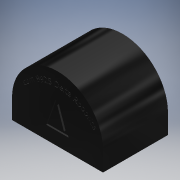
# Autodesk Inventor part: wheel cover
Saved by Autodesk Inventor 2019 (Build 230136000, 136)
## iProperties
Part Number: wheel cover
Material: Generic
Document SubType Name: Modeling
Designer: Delta
Appearance: Default(1)
Author: Delta
Autodesk Inventor part; units mm, degrees
ref_plane "YZ Plane" through (0, 0, 0) normal (1, 0, 0) x (0, 1, 0)
ref_plane "XZ Plane" through (0, 0, 0) normal (0, 1, 0) x (-1, 0, 0)
ref_plane "XY Plane" through (0, 0, 0) normal (0, 0, 1) x (1, 0, 0)
sketch "Sketch2" plane through (0, 0, 0) normal (0, 0, 1) x (1, 0, 0)
  circle A0 centre (0, 0) radius 44.45
  line L0 (44.45, 0) -> (-44.45, 0)
  dimension "d3" = 88.9
  constraints: 2 end point, 2 point on circle, 1 centre point, 1 coincident, 1 horizontal
  measures "d3" diameter of A0
extrude "Extrusion2" add sketch "Sketch2" along normal blind 63.5 contours L0 A0 picked at (-1.5488, 26.7885)
shell "Shell2" thickness 3.175 removed faces 1 at (4.5786, 14.0915, 0)
sketch "Sketch3" plane through (-44.45, 0, 0) normal (0, -1, 0) x (1, 0, 0)
  line L0 (3.2973, 0) -> (3.2973, 60.325) projected
  line L1 (3.2973, 60.325) -> (85.6027, 60.325) projected
  line L2 (85.6027, 0) -> (85.6027, 60.325) projected
  line L3 (0, 0) -> (88.9, 0) projected
  point P0 (44.45, 0)
extrude "Extrusion3" cut sketch "Sketch3" against normal blind 3.175
sketch "Sketch8" plane through (-44.45, 0, 63.5) normal (0, -1, 0) x (1, 0, 0)
  line L0 (3.2973, -63.5) -> (3.2973, -3.175) projected
  line L1 (3.2973, -3.175) -> (85.6027, -3.175) projected
  line L2 (85.6027, -3.175) -> (85.6027, -63.5) projected
  line L3 (85.6027, -63.5) -> (88.9, -63.5) projected
  line L4 (88.9, -63.5) -> (88.9, 0) projected
  line L5 (0, 0) -> (88.9, 0) projected
  line L6 (0, -63.5) -> (0, 0) projected
  line L7 (0, -63.5) -> (3.2973, -63.5) projected
  point P0 (44.45, -63.5)
extrude "Extrusion6" add sketch "Sketch8" along normal blind 19.05
sketch "Sketch15" plane through (0, 0, 63.5) normal (0, 0, 1) x (1, 0, 0)
  line L0 (-19.05, 19.05) -> (19.05, 19.05) construction
  line L1 (19.05, 19.05) -> (19.05, -6.35) construction
  line L2 (19.05, -6.35) -> (-19.05, -6.35) construction
  line L3 (-19.05, -6.35) -> (-19.05, 19.05) construction
  line L4 (44.45, -17.78) -> (44.45, 0) projected
  line L5 (-44.45, 0) -> (-44.45, -17.78) projected
  line L6 (-43.18, -19.05) -> (43.18, -19.05) projected
  line L7 (10.8166, -6.35) -> (-11.1459, -6.35)
  line L8 (-11.1459, -6.35) -> (-2.2539, 19.05)
  line L9 (-2.2539, 19.05) -> (1.9246, 19.05)
  line L10 (1.9246, 19.05) -> (10.8166, -6.35)
  line L11 (6.2677, -3.4271) -> (-0.2573, 15.7155)
  line L12 (-0.2573, 15.7155) -> (-6.7411, -3.4271)
  line L13 (-6.7411, -3.4271) -> (6.2677, -3.4271)
  point P0 (0, 0)
  dimension "d55" = 25.4
  dimension "d56" = 25.4
  dimension "d57" = 12.7
  dimension "d58" = 38.1
  constraints: 2 other
  measures "d55" distance between parallel lines of L4 L1
  measures "d56" distance between parallel lines of L5 L3
  measures "d57" distance between parallel lines of L6 L2
  measures "d58" distance between parallel lines of L6 L0
extrude "Extrusion10" cut sketch "Sketch15" against normal blind 1.5875
sketch "Sketch16" plane through (0, 0, 63.5) normal (0, 0, 1) x (1, 0, 0)
  line L0 (-44.45, 0) -> (-44.45, -17.78) projected
  line L1 (-43.18, 41.275) -> (-43.18, -17.78) projected
  arc A0 (42.9782, -8.89) -> (-43.18, -8.89) centre (-0.1009, -13.0404) ccw
  line L2 (-43.18, -8.89) -> (42.9782, -8.89) construction
  line L3 (-43.18, -8.89) -> (42.9782, -8.89) construction
  line L4 (-33.5603, 14.4116) -> (-37.0005, 17.2799)
  line L5 (-37.0005, 17.2799) -> (-38.0919, 15.9708)
  line L6 (-38.0919, 15.9708) -> (-38.5535, 16.3557)
  line L7 (-38.5535, 16.3557) -> (-35.9384, 19.4923)
  line L8 (-35.9384, 19.4923) -> (-35.4767, 19.1074)
  line L9 (-35.4767, 19.1074) -> (-36.5681, 17.7984)
  line L10 (-36.5681, 17.7984) -> (-33.128, 14.9302)
  line L11 (-33.128, 14.9302) -> (-33.5603, 14.4116)
  spline S0 degree 2 poles (-30.4682, 17.6755) (-31.1139, 17.0287) (-32.549, 17.0421) (-33.219, 17.7111) knots 0 0 0 1 2 2 2
  spline S1 degree 2 poles (-33.219, 17.7111) (-33.8774, 18.3684) (-33.9689, 19.8384) (-33.4134, 20.3948) knots 0 0 0 1 2 2 2
  spline S2 degree 2 poles (-33.4134, 20.3948) (-33.1632, 20.6454) (-32.6307, 20.8874) (-32.3338, 20.876) knots 0 0 0 1 2 2 2
  spline S3 degree 2 poles (-32.3338, 20.876) (-32.034, 20.8675) (-31.4341, 20.5769) (-31.1107, 20.2541) knots 0 0 0 1 2 2 2
  line L12 (-31.1107, 20.2541) -> (-30.863, 20.0068)
  line L13 (-30.863, 20.0068) -> (-32.7274, 18.1394)
  spline S4 degree 2 poles (-32.7274, 18.1394) (-32.2584, 17.6711) (-31.289, 17.6457) (-30.8702, 18.0652) knots 0 0 0 1 2 2 2
  spline S5 degree 2 poles (-30.8702, 18.0652) (-30.7219, 18.2138) (-30.5009, 18.5691) (-30.437, 18.738) knots 0 0 0 1 2 2 2
  spline S6 degree 2 poles (-30.437, 18.738) (-30.3731, 18.9185) (-30.3064, 19.1893) (-30.2977, 19.2912) knots 0 0 0 1 2 2 2
  line L14 (-30.2977, 19.2912) -> (-30.2716, 19.3174)
  line L15 (-30.2716, 19.3174) -> (-29.7763, 18.823)
  spline S7 degree 2 poles (-29.7763, 18.823) (-29.8228, 18.7123) (-29.9681, 18.3804) (-30.0349, 18.2609) knots 0 0 0 1 2 2 2
  spline S8 degree 2 poles (-30.0349, 18.2609) (-30.1279, 18.092) (-30.3053, 17.8386) (-30.4682, 17.6755) knots 0 0 0 1 2 2 2
  spline S9 degree 2 poles (-31.6518, 19.9101) (-31.8412, 20.0875) (-32.1848, 20.2794) (-32.3479, 20.2967) knots 0 0 0 1 2 2 2
  spline S10 degree 2 poles (-32.3479, 20.2967) (-32.5284, 20.3198) (-32.8834, 20.1798) (-33.0666, 19.9963) knots 0 0 0 1 2 2 2
  spline S11 degree 2 poles (-33.0666, 19.9963) (-33.247, 19.8157) (-33.3922, 19.4546) (-33.392, 19.245) knots 0 0 0 1 2 2 2
  spline S12 degree 2 poles (-33.392, 19.245) (-33.386, 19.0354) (-33.2315, 18.6717) (-33.0741, 18.4855) knots 0 0 0 1 2 2 2
  line L16 (-33.0741, 18.4855) -> (-31.6518, 19.9101)
  spline S13 degree 2 poles (-27.712, 20.8168) (-27.7346, 20.7223) (-27.803, 20.3951) (-27.8575, 20.2682) knots 0 0 0 1 2 2 2
  spline S14 degree 2 poles (-27.8575, 20.2682) (-27.928, 20.0901) (-28.1091, 19.8132) (-28.3292, 19.6273) knots 0 0 0 1 2 2 2
  spline S15 degree 2 poles (-28.3292, 19.6273) (-28.5085, 19.4758) (-28.9466, 19.3374) (-29.1729, 19.3565) knots 0 0 0 1 2 2 2
  spline S16 degree 2 poles (-29.1729, 19.3565) (-29.3902, 19.3777) (-29.8292, 19.6104) (-29.9939, 19.8054) knots 0 0 0 1 2 2 2
  spline S17 degree 2 poles (-29.9939, 19.8054) (-30.249, 20.1073) (-30.3555, 20.7501) (-30.1824, 21.1066) knots 0 0 0 1 2 2 2
  spline S18 degree 2 poles (-30.1824, 21.1066) (-30.0327, 21.427) (-29.4377, 22.0751) (-29.0695, 22.4238) knots 0 0 0 1 2 2 2
  line L17 (-29.0695, 22.4238) -> (-29.1492, 22.5182)
  spline S19 degree 2 poles (-29.1492, 22.5182) (-29.2926, 22.688) (-29.5744, 22.8111) (-29.7192, 22.7911) knots 0 0 0 1 2 2 2
  spline S20 degree 2 poles (-29.7192, 22.7911) (-29.8641, 22.7712) (-30.1664, 22.5804) (-30.311, 22.4582) knots 0 0 0 1 2 2 2
  spline S21 degree 2 poles (-30.311, 22.4582) (-30.4809, 22.3148) (-30.855, 21.8263) (-31.0022, 21.5349) knots 0 0 0 1 2 2 2
  line L18 (-31.0022, 21.5349) -> (-31.0305, 21.511)
  line L19 (-31.0305, 21.511) -> (-31.4529, 22.011)
  spline S22 degree 2 poles (-31.4529, 22.011) (-31.3496, 22.163) (-30.9229, 22.685) (-30.6745, 22.8949) knots 0 0 0 1 2 2 2
  spline S23 degree 2 poles (-30.6745, 22.8949) (-30.3726, 23.1499) (-29.8809, 23.4036) (-29.6138, 23.4191) knots 0 0 0 1 2 2 2
  spline S24 degree 2 poles (-29.6138, 23.4191) (-29.3525, 23.435) (-28.8738, 23.1873) (-28.6427, 22.9137) knots 0 0 0 1 2 2 2
  line L20 (-28.6427, 22.9137) -> (-26.9611, 20.923)
  line L21 (-26.9611, 20.923) -> (-27.4517, 20.5086)
  line L22 (-27.4517, 20.5086) -> (-27.712, 20.8168)
  line L23 (-28.0574, 21.2257) -> (-28.7401, 22.0339)
  spline S25 degree 2 poles (-28.7401, 22.0339) (-28.9029, 21.8694) (-29.3892, 21.367) (-29.5134, 21.1759) knots 0 0 0 1 2 2 2
  spline S26 degree 2 poles (-29.5134, 21.1759) (-29.6579, 20.9514) (-29.7028, 20.4878) (-29.5168, 20.2677) knots 0 0 0 1 2 2 2
  spline S27 degree 2 poles (-29.5168, 20.2677) (-29.3043, 20.0161) (-28.8061, 20.0004) (-28.5356, 20.2289) knots 0 0 0 1 2 2 2
  spline S28 degree 2 poles (-28.5356, 20.2289) (-28.3061, 20.4228) (-28.096, 20.9397) (-28.0574, 21.2257) knots 0 0 0 1 2 2 2
  line L24 (-22.6902, 23.9217) -> (-23.9204, 25.7535)
  spline S29 degree 2 poles (-23.9204, 25.7535) (-24.0673, 25.9722) (-24.3516, 26.3218) (-24.4751, 26.3876) knots 0 0 0 1 2 2 2
  spline S30 degree 2 poles (-24.4751, 26.3876) (-24.6056, 26.4636) (-24.8875, 26.433) (-25.0686, 26.3113) knots 0 0 0 1 2 2 2
  spline S31 degree 2 poles (-25.0686, 26.3113) (-25.2326, 26.2012) (-25.4732, 25.7471) (-25.5428, 25.4226) knots 0 0 0 1 2 2 2
  spline S32 degree 2 poles (-25.5428, 25.4226) (-25.5073, 25.377) (-25.4109, 25.2483) (-25.3513, 25.1595) knots 0 0 0 1 2 2 2
  line L25 (-25.3513, 25.1595) -> (-23.9512, 23.0748)
  line L26 (-23.9512, 23.0748) -> (-24.4844, 22.7167)
  line L27 (-24.4844, 22.7167) -> (-25.7146, 24.5485)
  spline S33 degree 2 poles (-25.7146, 24.5485) (-25.8615, 24.7672) (-26.1458, 25.1168) (-26.2693, 25.1826) knots 0 0 0 1 2 2 2
  spline S34 degree 2 poles (-26.2693, 25.1826) (-26.3998, 25.2587) (-26.6817, 25.228) (-26.8628, 25.1064) knots 0 0 0 1 2 2 2
  spline S35 degree 2 poles (-26.8628, 25.1064) (-27.0337, 24.9916) (-27.2684, 24.5215) (-27.3337, 24.2347) knots 0 0 0 1 2 2 2
  line L28 (-27.3337, 24.2347) -> (-25.7454, 21.8698)
  line L29 (-25.7454, 21.8698) -> (-26.2786, 21.5118)
  line L30 (-26.2786, 21.5118) -> (-28.4039, 24.6764)
  line L31 (-28.4039, 24.6764) -> (-27.8707, 25.0344)
  line L32 (-27.8707, 25.0344) -> (-27.6366, 24.6859)
  spline S36 degree 2 poles (-27.6366, 24.6859) (-27.5682, 25.0343) (-27.3118, 25.5387) (-27.0658, 25.704) knots 0 0 0 1 2 2 2
  spline S37 degree 2 poles (-27.0658, 25.704) (-26.7855, 25.8922) (-26.1794, 25.9273) (-25.8715, 25.7126) knots 0 0 0 1 2 2 2
  spline S38 degree 2 poles (-25.8715, 25.7126) (-25.8102, 26.1455) (-25.5382, 26.7299) (-25.2716, 26.9089) knots 0 0 0 1 2 2 2
  spline S39 degree 2 poles (-25.2716, 26.9089) (-25.0665, 27.0466) (-24.6467, 27.1451) (-24.4273, 27.0842) knots 0 0 0 1 2 2 2
  spline S40 degree 2 poles (-24.4273, 27.0842) (-24.2044, 27.0256) (-23.7751, 26.6891) (-23.5571, 26.3644) knots 0 0 0 1 2 2 2
  line L33 (-23.5571, 26.3644) -> (-22.157, 24.2797)
  line L34 (-22.157, 24.2797) -> (-22.6902, 23.9217)
  spline S41 degree 2 poles (-21.0664, 28.7312) (-21.2291, 29.0868) (-21.2678, 29.7845) (-21.1634, 30.0904) knots 0 0 0 1 2 2 2
  spline S42 degree 2 poles (-21.1634, 30.0904) (-21.0667, 30.3836) (-20.6135, 30.8673) (-20.329, 30.9975) knots 0 0 0 1 2 2 2
  spline S43 degree 2 poles (-20.329, 30.9975) (-20.0109, 31.1432) (-19.3966, 31.1663) (-19.1132, 31.0516) knots 0 0 0 1 2 2 2
  spline S44 degree 2 poles (-19.1132, 31.0516) (-18.7571, 30.9067) (-18.1181, 30.2032) (-17.8285, 29.5706) knots 0 0 0 1 2 2 2
  spline S45 degree 2 poles (-17.8285, 29.5706) (-17.5664, 28.9979) (-17.3551, 27.854) (-17.45, 27.3986) knots 0 0 0 1 2 2 2
  spline S46 degree 2 poles (-17.45, 27.3986) (-17.5512, 26.9176) (-18.1268, 26.1968) (-18.6733, 25.9466) knots 0 0 0 1 2 2 2
  spline S47 degree 2 poles (-18.6733, 25.9466) (-18.7968, 25.8901) (-19.0895, 25.7878) (-19.2264, 25.7704) knots 0 0 0 1 2 2 2
  line L35 (-19.2264, 25.7704) -> (-19.4989, 26.3655)
  line L36 (-19.4989, 26.3655) -> (-19.469, 26.3792)
  spline S48 degree 2 poles (-19.469, 26.3792) (-19.3698, 26.3703) (-19.0044, 26.4425) (-18.836, 26.5196) knots 0 0 0 1 2 2 2
  spline S49 degree 2 poles (-18.836, 26.5196) (-18.2296, 26.7972) (-17.9038, 27.9152) (-18.1944, 28.6787) knots 0 0 0 1 2 2 2
  spline S50 degree 2 poles (-18.1944, 28.6787) (-18.3644, 28.3971) (-18.7433, 28.038) (-19.0091, 27.9164) knots 0 0 0 1 2 2 2
  spline S51 degree 2 poles (-19.0091, 27.9164) (-19.2636, 27.7998) (-19.738, 27.7185) (-20.025, 27.7818) knots 0 0 0 1 2 2 2
  spline S52 degree 2 poles (-20.025, 27.7818) (-20.3594, 27.8596) (-20.8796, 28.3232) (-21.0664, 28.7312) knots 0 0 0 1 2 2 2
  spline S53 degree 2 poles (-18.517, 29.4229) (-18.7312, 29.8908) (-19.1742, 30.4034) (-19.4013, 30.4941) knots 0 0 0 1 2 2 2
  spline S54 degree 2 poles (-19.4013, 30.4941) (-19.6046, 30.5821) (-19.9367, 30.5659) (-20.1014, 30.4905) knots 0 0 0 1 2 2 2
  spline S55 degree 2 poles (-20.1014, 30.4905) (-20.4832, 30.3157) (-20.686, 29.5619) (-20.4495, 29.0453) knots 0 0 0 1 2 2 2
  spline S56 degree 2 poles (-20.4495, 29.0453) (-20.3158, 28.7534) (-19.9931, 28.4438) (-19.7667, 28.3845) knots 0 0 0 1 2 2 2
  spline S57 degree 2 poles (-19.7667, 28.3845) (-19.6023, 28.342) (-19.2775, 28.4137) (-19.1053, 28.4926) knots 0 0 0 1 2 2 2
  spline S58 degree 2 poles (-19.1053, 28.4926) (-18.9069, 28.5834) (-18.5137, 28.9309) (-18.3946, 29.1258) knots 0 0 0 1 2 2 2
  spline S59 degree 2 poles (-18.3946, 29.1258) (-18.4114, 29.1724) (-18.4742, 29.3293) (-18.517, 29.4229) knots 0 0 0 1 2 2 2
  spline S60 degree 2 poles (-17.313, 30.4126) (-17.4439, 30.7811) (-17.4211, 31.4795) (-17.2901, 31.775) knots 0 0 0 1 2 2 2
  spline S61 degree 2 poles (-17.2901, 31.775) (-17.1681, 32.0586) (-16.6741, 32.5006) (-16.3793, 32.6053) knots 0 0 0 1 2 2 2
  spline S62 degree 2 poles (-16.3793, 32.6053) (-16.0495, 32.7224) (-15.4357, 32.6914) (-15.1634, 32.5522) knots 0 0 0 1 2 2 2
  spline S63 degree 2 poles (-15.1634, 32.5522) (-14.8214, 32.3766) (-14.2468, 31.6196) (-14.0139, 30.9641) knots 0 0 0 1 2 2 2
  spline S64 degree 2 poles (-14.0139, 30.9641) (-13.8031, 30.3705) (-13.6932, 29.2125) (-13.8278, 28.7672) knots 0 0 0 1 2 2 2
  spline S65 degree 2 poles (-13.8278, 28.7672) (-13.9709, 28.297) (-14.6076, 27.6296) (-15.174, 27.4284) knots 0 0 0 1 2 2 2
  spline S66 degree 2 poles (-15.174, 27.4284) (-15.302, 27.383) (-15.6026, 27.3068) (-15.7405, 27.3015) knots 0 0 0 1 2 2 2
  line L37 (-15.7405, 27.3015) -> (-15.9596, 27.9183)
  line L38 (-15.9596, 27.9183) -> (-15.9285, 27.9293)
  spline S67 degree 2 poles (-15.9285, 27.9293) (-15.8305, 27.9117) (-15.4602, 27.9515) (-15.2857, 28.0135) knots 0 0 0 1 2 2 2
  spline S68 degree 2 poles (-15.2857, 28.0135) (-14.6572, 28.2367) (-14.2344, 29.3217) (-14.4568, 30.1078) knots 0 0 0 1 2 2 2
  spline S69 degree 2 poles (-14.4568, 30.1078) (-14.6508, 29.8422) (-15.0598, 29.5179) (-15.3353, 29.42) knots 0 0 0 1 2 2 2
  spline S70 degree 2 poles (-15.3353, 29.42) (-15.5991, 29.3263) (-16.0788, 29.287) (-16.3591, 29.3753) knots 0 0 0 1 2 2 2
  spline S71 degree 2 poles (-16.3591, 29.3753) (-16.6854, 29.4822) (-17.1628, 29.9898) (-17.313, 30.4126) knots 0 0 0 1 2 2 2
  spline S72 degree 2 poles (-14.7127, 30.8775) (-14.885, 31.3624) (-15.2811, 31.9119) (-15.4994, 32.0222) knots 0 0 0 1 2 2 2
  spline S73 degree 2 poles (-15.4994, 32.0222) (-15.6942, 32.1278) (-16.0265, 32.1408) (-16.1971, 32.0802) knots 0 0 0 1 2 2 2
  spline S74 degree 2 poles (-16.1971, 32.0802) (-16.5928, 31.9397) (-16.861, 31.2066) (-16.6709, 30.6712) knots 0 0 0 1 2 2 2
  spline S75 degree 2 poles (-16.6709, 30.6712) (-16.5634, 30.3687) (-16.2691, 30.032) (-16.0488, 29.9529) knots 0 0 0 1 2 2 2
  spline S76 degree 2 poles (-16.0488, 29.9529) (-15.8888, 29.8962) (-15.559, 29.9391) (-15.3805, 30.0025) knots 0 0 0 1 2 2 2
  spline S77 degree 2 poles (-15.3805, 30.0025) (-15.1749, 30.0755) (-14.7526, 30.3871) (-14.6169, 30.5708) knots 0 0 0 1 2 2 2
  spline S78 degree 2 poles (-14.6169, 30.5708) (-14.6295, 30.6187) (-14.6783, 30.7805) (-14.7127, 30.8775) knots 0 0 0 1 2 2 2
  line L39 (-9.3987, 29.2577) -> (-12.4316, 28.4728)
  line L40 (-12.4316, 28.4728) -> (-12.6121, 29.1702)
  spline S79 degree 2 poles (-12.6121, 29.1702) (-12.3647, 29.5617) (-11.9304, 30.2822) (-11.7308, 30.6613) knots 0 0 0 1 2 2 2
  spline S80 degree 2 poles (-11.7308, 30.6613) (-11.3287, 31.4244) (-11.1101, 32.2719) (-11.2122, 32.6665) knots 0 0 0 1 2 2 2
  spline S81 degree 2 poles (-11.2122, 32.6665) (-11.2659, 32.8737) (-11.4739, 33.1516) (-11.6152, 33.2213) knots 0 0 0 1 2 2 2
  spline S82 degree 2 poles (-11.6152, 33.2213) (-11.7566, 33.291) (-12.0853, 33.3123) (-12.2686, 33.2648) knots 0 0 0 1 2 2 2
  spline S83 degree 2 poles (-12.2686, 33.2648) (-12.4439, 33.2194) (-12.7799, 33.0389) (-12.9258, 32.9289) knots 0 0 0 1 2 2 2
  spline S84 degree 2 poles (-12.9258, 32.9289) (-13.0508, 32.837) (-13.2686, 32.6105) (-13.3339, 32.5341) knots 0 0 0 1 2 2 2
  line L41 (-13.3339, 32.5341) -> (-13.3698, 32.5248)
  line L42 (-13.3698, 32.5248) -> (-13.5513, 33.2262)
  spline S85 degree 2 poles (-13.5513, 33.2262) (-13.3738, 33.3785) (-12.6951, 33.7625) (-12.3683, 33.8471) knots 0 0 0 1 2 2 2
  spline S86 degree 2 poles (-12.3683, 33.8471) (-11.6788, 34.0256) (-10.7129, 33.4974) (-10.552, 32.8757) knots 0 0 0 1 2 2 2
  spline S87 degree 2 poles (-10.552, 32.8757) (-10.4767, 32.5847) (-10.4863, 32.0634) (-10.5523, 31.8253) knots 0 0 0 1 2 2 2
  spline S88 degree 2 poles (-10.5523, 31.8253) (-10.6161, 31.5791) (-10.8535, 31.0669) (-10.9922, 30.8141) knots 0 0 0 1 2 2 2
  spline S89 degree 2 poles (-10.9922, 30.8141) (-11.2154, 30.3949) (-11.7888, 29.4726) (-11.9613, 29.2026) knots 0 0 0 1 2 2 2
  line L43 (-11.9613, 29.2026) -> (-9.5462, 29.8277)
  line L44 (-9.5462, 29.8277) -> (-9.3987, 29.2577)
  spline S90 degree 2 poles (-5.9624, 31.4943) (-5.9022, 31.1329) (-6.0307, 30.4771) (-6.2039, 30.2145) knots 0 0 0 1 2 2 2
  spline S91 degree 2 poles (-6.2039, 30.2145) (-6.3772, 29.9519) (-6.9626, 29.583) (-7.3524, 29.518) knots 0 0 0 1 2 2 2
  spline S92 degree 2 poles (-7.3524, 29.518) (-7.7097, 29.4584) (-8.4345, 29.5003) (-8.7114, 29.5835) knots 0 0 0 1 2 2 2
  line L45 (-8.7114, 29.5835) -> (-8.8299, 30.2941)
  line L46 (-8.8299, 30.2941) -> (-8.7811, 30.3023)
  spline S93 degree 2 poles (-8.7811, 30.3023) (-8.6945, 30.2583) (-8.3818, 30.1602) (-8.1964, 30.1243) knots 0 0 0 1 2 2 2
  spline S94 degree 2 poles (-8.1964, 30.1243) (-7.9859, 30.0885) (-7.6441, 30.0662) (-7.437, 30.1007) knots 0 0 0 1 2 2 2
  spline S95 degree 2 poles (-7.437, 30.1007) (-7.234, 30.1346) (-6.8767, 30.3444) (-6.765, 30.5258) knots 0 0 0 1 2 2 2
  spline S96 degree 2 poles (-6.765, 30.5258) (-6.6642, 30.697) (-6.6006, 31.1166) (-6.6453, 31.3846) knots 0 0 0 1 2 2 2
  spline S97 degree 2 poles (-6.6453, 31.3846) (-6.69, 31.6526) (-6.8931, 31.9693) (-7.0501, 32.06) knots 0 0 0 1 2 2 2
  spline S98 degree 2 poles (-7.0501, 32.06) (-7.2132, 32.1622) (-7.6531, 32.1973) (-7.9089, 32.1547) knots 0 0 0 1 2 2 2
  spline S99 degree 2 poles (-7.9089, 32.1547) (-8.185, 32.1086) (-8.719, 31.9319) (-8.8794, 31.8676) knots 0 0 0 1 2 2 2
  line L47 (-8.8794, 31.8676) -> (-9.3101, 34.4502)
  line L48 (-9.3101, 34.4502) -> (-6.561, 34.9086)
  line L49 (-6.561, 34.9086) -> (-6.4628, 34.3198)
  line L50 (-6.4628, 34.3198) -> (-8.5662, 33.9691)
  line L51 (-8.5662, 33.9691) -> (-8.3435, 32.6331)
  spline S100 degree 2 poles (-8.3435, 32.6331) (-8.2244, 32.6697) (-7.9909, 32.7211) (-7.8934, 32.7374) knots 0 0 0 1 2 2 2
  spline S101 degree 2 poles (-7.8934, 32.7374) (-7.5077, 32.8017) (-6.9547, 32.7645) (-6.6799, 32.6184) knots 0 0 0 1 2 2 2
  spline S102 degree 2 poles (-6.6799, 32.6184) (-6.4011, 32.4729) (-6.0383, 31.9491) (-5.9624, 31.4943) knots 0 0 0 1 2 2 2
  spline S103 degree 2 poles (1.3105, 32.8027) (1.3218, 32.1071) (0.7759, 30.9784) (0.3076, 30.658) knots 0 0 0 1 2 2 2
  spline S104 degree 2 poles (0.3076, 30.658) (-0.0754, 30.4089) (-0.8671, 30.2314) (-1.4846, 30.2214) knots 0 0 0 1 2 2 2
  line L52 (-1.4846, 30.2214) -> (-2.6536, 30.2026)
  line L53 (-2.6536, 30.2026) -> (-2.7355, 35.2819)
  line L54 (-2.7355, 35.2819) -> (-1.5789, 35.3006)
  spline S105 degree 2 poles (-1.5789, 35.3006) (-0.8627, 35.3121) (-0.0442, 35.1112) (0.247, 34.9265) knots 0 0 0 1 2 2 2
  spline S106 degree 2 poles (0.247, 34.9265) (0.742, 34.6093) (1.2986, 33.5437) (1.3105, 32.8027) knots 0 0 0 1 2 2 2
  spline S107 degree 2 poles (0.6066, 32.7996) (0.5971, 33.3841) (0.1969, 34.2052) (-0.1897, 34.4337) knots 0 0 0 1 2 2 2
  spline S108 degree 2 poles (-0.1897, 34.4337) (-0.464, 34.5898) (-1.0796, 34.724) (-1.5365, 34.7166) knots 0 0 0 1 2 2 2
  line L55 (-1.5365, 34.7166) -> (-2.051, 34.7083)
  line L56 (-2.051, 34.7083) -> (-1.9879, 30.798)
  line L57 (-1.9879, 30.798) -> (-1.4734, 30.8063)
  spline S109 degree 2 poles (-1.4734, 30.8063) (-1.0248, 30.8135) (-0.3479, 30.9685) (-0.0753, 31.1664) knots 0 0 0 1 2 2 2
  spline S110 degree 2 poles (-0.0753, 31.1664) (0.2749, 31.4109) (0.6161, 32.2069) (0.6066, 32.7996) knots 0 0 0 1 2 2 2
  spline S111 degree 2 poles (3.6748, 29.9873) (2.7639, 30.0612) (1.8456, 31.1642) (1.9222, 32.1079) knots 0 0 0 1 2 2 2
  spline S112 degree 2 poles (1.9222, 32.1079) (1.9975, 33.0352) (3.0592, 34.0559) (3.8429, 33.9923) knots 0 0 0 1 2 2 2
  spline S113 degree 2 poles (3.8429, 33.9923) (4.1958, 33.9637) (4.7249, 33.7142) (4.9083, 33.4804) knots 0 0 0 1 2 2 2
  spline S114 degree 2 poles (4.9083, 33.4804) (5.0958, 33.2463) (5.2623, 32.6009) (5.2253, 32.1454) knots 0 0 0 1 2 2 2
  line L58 (5.2253, 32.1454) -> (5.197, 31.7966)
  line L59 (5.197, 31.7966) -> (2.5669, 32.0101)
  spline S115 degree 2 poles (2.5669, 32.0101) (2.5133, 31.3495) (3.121, 30.5939) (3.7119, 30.546) knots 0 0 0 1 2 2 2
  spline S116 degree 2 poles (3.7119, 30.546) (3.9211, 30.529) (4.335, 30.5904) (4.5051, 30.6509) knots 0 0 0 1 2 2 2
  spline S117 degree 2 poles (4.5051, 30.6509) (4.6841, 30.719) (4.9338, 30.8433) (5.0171, 30.9026) knots 0 0 0 1 2 2 2
  line L60 (5.0171, 30.9026) -> (5.054, 30.8996)
  line L61 (5.054, 30.8996) -> (4.9974, 30.202)
  spline S118 degree 2 poles (4.9974, 30.202) (4.8829, 30.1659) (4.5358, 30.0619) (4.4015, 30.0356) knots 0 0 0 1 2 2 2
  spline S119 degree 2 poles (4.4015, 30.0356) (4.2125, 29.9973) (3.9046, 29.9686) (3.6748, 29.9873) knots 0 0 0 1 2 2 2
  spline S120 degree 2 poles (4.613, 32.3355) (4.6258, 32.5947) (4.5497, 32.9809) (4.4575, 33.1164) knots 0 0 0 1 2 2 2
  spline S121 degree 2 poles (4.4575, 33.1164) (4.3583, 33.269) (4.0219, 33.4491) (3.7634, 33.4701) knots 0 0 0 1 2 2 2
  spline S122 degree 2 poles (3.7634, 33.4701) (3.509, 33.4908) (3.1397, 33.3679) (2.98, 33.2322) knots 0 0 0 1 2 2 2
  spline S123 degree 2 poles (2.98, 33.2322) (2.824, 33.092) (2.6467, 32.7388) (2.6065, 32.4984) knots 0 0 0 1 2 2 2
  line L62 (2.6065, 32.4984) -> (4.613, 32.3355)
  line L63 (6.3374, 29.7578) -> (5.7016, 29.8486)
  line L64 (5.7016, 29.8486) -> (6.4521, 35.1017)
  line L65 (6.4521, 35.1017) -> (7.0878, 35.0108)
  line L66 (7.0878, 35.0108) -> (6.3374, 29.7578)
  spline S124 degree 2 poles (8.3872, 29.3244) (7.8735, 29.4218) (7.4063, 30.1179) (7.5267, 30.7529) knots 0 0 0 1 2 2 2
  line L67 (7.5267, 30.7529) -> (7.9201, 32.8278)
  line L68 (7.9201, 32.8278) -> (7.4954, 32.9083)
  line L69 (7.4954, 32.9083) -> (7.5943, 33.4301)
  line L70 (7.5943, 33.4301) -> (8.019, 33.3496)
  line L71 (8.019, 33.3496) -> (8.2229, 34.4254)
  line L72 (8.2229, 34.4254) -> (8.8539, 34.3058)
  line L73 (8.8539, 34.3058) -> (8.6499, 33.23)
  line L74 (8.6499, 33.23) -> (9.8108, 33.0099)
  line L75 (9.8108, 33.0099) -> (9.7118, 32.4881)
  line L76 (9.7118, 32.4881) -> (8.551, 32.7082)
  line L77 (8.551, 32.7082) -> (8.2129, 30.9245)
  spline S125 degree 2 poles (8.2129, 30.9245) (8.1592, 30.6414) (8.1204, 30.3261) (8.1638, 30.1796) knots 0 0 0 1 2 2 2
  spline S126 degree 2 poles (8.1638, 30.1796) (8.1982, 30.0516) (8.4308, 29.886) (8.6492, 29.8446) knots 0 0 0 1 2 2 2
  spline S127 degree 2 poles (8.6492, 29.8446) (8.8029, 29.8154) (9.1077, 29.854) (9.1778, 29.8701) knots 0 0 0 1 2 2 2
  line L78 (9.1778, 29.8701) -> (9.2142, 29.8631)
  line L79 (9.2142, 29.8631) -> (9.1069, 29.2969)
  spline S128 degree 2 poles (9.1069, 29.2969) (8.9197, 29.2821) (8.5449, 29.2945) (8.3872, 29.3244) knots 0 0 0 1 2 2 2
  spline S129 degree 2 poles (11.7207, 29.0183) (11.6304, 28.9824) (11.3233, 28.8502) (11.1882, 28.8218) knots 0 0 0 1 2 2 2
  spline S130 degree 2 poles (11.1882, 28.8218) (11.0019, 28.7771) (10.6713, 28.766) (10.3926, 28.8392) knots 0 0 0 1 2 2 2
  spline S131 degree 2 poles (10.3926, 28.8392) (10.1656, 28.8987) (9.8004, 29.1776) (9.6859, 29.3737) knots 0 0 0 1 2 2 2
  spline S132 degree 2 poles (9.6859, 29.3737) (9.5783, 29.5637) (9.5162, 30.0567) (9.581, 30.3035) knots 0 0 0 1 2 2 2
  spline S133 degree 2 poles (9.581, 30.3035) (9.6813, 30.6858) (10.146, 31.1426) (10.5372, 31.2059) knots 0 0 0 1 2 2 2
  spline S134 degree 2 poles (10.5372, 31.2059) (10.8854, 31.2678) (11.7577, 31.1537) (12.2548, 31.053) knots 0 0 0 1 2 2 2
  line L80 (12.2548, 31.053) -> (12.2862, 31.1724)
  spline S135 degree 2 poles (12.2862, 31.1724) (12.3426, 31.3875) (12.2813, 31.6887) (12.1817, 31.7957) knots 0 0 0 1 2 2 2
  spline S136 degree 2 poles (12.1817, 31.7957) (12.0821, 31.9028) (11.7522, 32.0404) (11.569, 32.0885) knots 0 0 0 1 2 2 2
  spline S137 degree 2 poles (11.569, 32.0885) (11.354, 32.1449) (10.7392, 32.1701) (10.4161, 32.123) knots 0 0 0 1 2 2 2
  line L81 (10.4161, 32.123) -> (10.3803, 32.1324)
  line L82 (10.3803, 32.1324) -> (10.5465, 32.7655)
  spline S138 degree 2 poles (10.5465, 32.7655) (10.7302, 32.7684) (11.4027, 32.7195) (11.7172, 32.6369) knots 0 0 0 1 2 2 2
  spline S139 degree 2 poles (11.7172, 32.6369) (12.0995, 32.5366) (12.5897, 32.2802) (12.756, 32.0706) knots 0 0 0 1 2 2 2
  spline S140 degree 2 poles (12.756, 32.0706) (12.9194, 31.866) (12.992, 31.3319) (12.9011, 30.9855) knots 0 0 0 1 2 2 2
  line L83 (12.9011, 30.9855) -> (12.2394, 28.465)
  line L84 (12.2394, 28.465) -> (11.6183, 28.6281)
  line L85 (11.6183, 28.6281) -> (11.7207, 29.0183)
  line L86 (11.8566, 29.5359) -> (12.1252, 30.5592)
  spline S141 degree 2 poles (12.1252, 30.5592) (11.897, 30.5979) (11.2063, 30.7068) (10.9786, 30.6985) knots 0 0 0 1 2 2 2
  spline S142 degree 2 poles (10.9786, 30.6985) (10.7118, 30.6877) (10.3067, 30.4578) (10.2336, 30.179) knots 0 0 0 1 2 2 2
  spline S143 degree 2 poles (10.2336, 30.179) (10.1499, 29.8605) (10.4236, 29.4439) (10.7661, 29.354) knots 0 0 0 1 2 2 2
  spline S144 degree 2 poles (10.7661, 29.354) (11.0567, 29.2777) (11.6004, 29.4031) (11.8566, 29.5359) knots 0 0 0 1 2 2 2
  line L87 (18.832, 25.9438) -> (18.0242, 26.2848)
  line L88 (18.0242, 26.2848) -> (17.3314, 28.7715)
  line L89 (17.3314, 28.7715) -> (16.6184, 29.0725)
  line L90 (16.6184, 29.0725) -> (15.8321, 27.2104)
  line L91 (15.8321, 27.2104) -> (15.2102, 27.473)
  line L92 (15.2102, 27.473) -> (17.1861, 32.1529)
  line L93 (17.1861, 32.1529) -> (18.3921, 31.6437)
  spline S145 degree 2 poles (18.3921, 31.6437) (18.7941, 31.474) (19.2996, 31.1578) (19.4789, 30.8944) knots 0 0 0 1 2 2 2
  spline S146 degree 2 poles (19.4789, 30.8944) (19.6582, 30.6311) (19.7328, 30.0142) (19.5775, 29.6463) knots 0 0 0 1 2 2 2
  spline S147 degree 2 poles (19.5775, 29.6463) (19.3613, 29.1343) (18.545, 28.6612) (18.027, 28.6833) knots 0 0 0 1 2 2 2
  line L94 (18.027, 28.6833) -> (18.832, 25.9438)
  spline S148 degree 2 poles (18.9082, 29.8708) (18.9946, 30.0756) (18.9834, 30.4512) (18.875, 30.6177) knots 0 0 0 1 2 2 2
  spline S149 degree 2 poles (18.875, 30.6177) (18.7791, 30.7609) (18.4568, 30.9819) (18.1989, 31.0908) knots 0 0 0 1 2 2 2
  line L95 (18.1989, 31.0908) -> (17.5807, 31.3518)
  line L96 (17.5807, 31.3518) -> (16.8377, 29.5921)
  line L97 (16.8377, 29.5921) -> (17.3839, 29.3615)
  spline S150 degree 2 poles (17.3839, 29.3615) (17.6531, 29.2478) (18.1217, 29.1617) (18.3321, 29.2471) knots 0 0 0 1 2 2 2
  spline S151 degree 2 poles (18.3321, 29.2471) (18.523, 29.3184) (18.8057, 29.6281) (18.9082, 29.8708) knots 0 0 0 1 2 2 2
  spline S152 degree 2 poles (22.7957, 25.9505) (22.3395, 25.102) (21.0266, 24.6161) (20.3449, 24.9826) knots 0 0 0 1 2 2 2
  spline S153 degree 2 poles (20.3449, 24.9826) (19.6451, 25.3588) (19.3565, 26.7432) (19.7971, 27.5627) knots 0 0 0 1 2 2 2
  spline S154 degree 2 poles (19.7971, 27.5627) (20.2494, 28.4039) (21.5771, 28.8912) (22.2515, 28.5286) knots 0 0 0 1 2 2 2
  spline S155 degree 2 poles (22.2515, 28.5286) (22.9332, 28.1621) (23.2499, 26.7953) (22.7957, 25.9505) knots 0 0 0 1 2 2 2
  spline S156 degree 2 poles (22.2119, 26.2643) (22.5628, 26.917) (22.429, 27.8069) (21.9903, 28.0428) knots 0 0 0 1 2 2 2
  spline S157 degree 2 poles (21.9903, 28.0428) (21.5515, 28.2787) (20.7318, 27.9015) (20.3809, 27.2488) knots 0 0 0 1 2 2 2
  spline S158 degree 2 poles (20.3809, 27.2488) (20.0397, 26.6143) (20.1674, 25.7043) (20.6062, 25.4684) knots 0 0 0 1 2 2 2
  spline S159 degree 2 poles (20.6062, 25.4684) (21.0413, 25.2345) (21.8649, 25.6189) (22.2119, 26.2643) knots 0 0 0 1 2 2 2
  spline S160 degree 2 poles (26.2033, 23.8148) (25.6899, 23.034) (24.3066, 22.5788) (23.7356, 22.9543) knots 0 0 0 1 2 2 2
  spline S161 degree 2 poles (23.7356, 22.9543) (23.4777, 23.1239) (23.1933, 23.4932) (23.0868, 23.7209) knots 0 0 0 1 2 2 2
  line L98 (23.0868, 23.7209) -> (22.9552, 23.5956)
  line L99 (22.9552, 23.5956) -> (22.453, 23.9258)
  line L100 (22.453, 23.9258) -> (25.3685, 28.3596)
  line L101 (25.3685, 28.3596) -> (25.905, 28.0067)
  line L102 (25.905, 28.0067) -> (24.8646, 26.4245)
  spline S162 degree 2 poles (24.8646, 26.4245) (25.1874, 26.4733) (25.817, 26.4042) (26.1162, 26.2074) knots 0 0 0 1 2 2 2
  spline S163 degree 2 poles (26.1162, 26.2074) (26.6563, 25.8523) (26.7077, 24.5819) (26.2033, 23.8148) knots 0 0 0 1 2 2 2
  spline S164 degree 2 poles (25.6224, 24.1377) (25.9978, 24.7087) (26.0395, 25.5287) (25.6542, 25.7821) knots 0 0 0 1 2 2 2
  spline S165 degree 2 poles (25.6542, 25.7821) (25.4375, 25.9246) (24.8547, 26.0122) (24.5683, 25.9739) knots 0 0 0 1 2 2 2
  line L103 (24.5683, 25.9739) -> (23.3673, 24.1474)
  spline S166 degree 2 poles (23.3673, 24.1474) (23.5046, 23.9142) (23.7634, 23.6258) (23.9491, 23.5037) knots 0 0 0 1 2 2 2
  spline S167 degree 2 poles (23.9491, 23.5037) (24.3584, 23.2345) (25.2085, 23.5082) (25.6224, 24.1377) knots 0 0 0 1 2 2 2
  spline S168 degree 2 poles (29.2936, 21.3181) (28.6953, 20.5631) (27.3174, 20.3155) (26.7108, 20.7961) knots 0 0 0 1 2 2 2
  spline S169 degree 2 poles (26.7108, 20.7961) (26.0881, 21.2895) (26.0473, 22.7031) (26.6251, 23.4324) knots 0 0 0 1 2 2 2
  spline S170 degree 2 poles (26.6251, 23.4324) (27.2182, 24.1809) (28.6109, 24.4273) (29.2111, 23.9518) knots 0 0 0 1 2 2 2
  spline S171 degree 2 poles (29.2111, 23.9518) (29.8177, 23.4712) (29.8892, 22.0699) (29.2936, 21.3181) knots 0 0 0 1 2 2 2
  spline S172 degree 2 poles (28.7741, 21.7297) (29.2342, 22.3105) (29.2589, 23.2101) (28.8685, 23.5194) knots 0 0 0 1 2 2 2
  spline S173 degree 2 poles (28.8685, 23.5194) (28.4781, 23.8288) (27.6048, 23.6016) (27.1446, 23.0208) knots 0 0 0 1 2 2 2
  spline S174 degree 2 poles (27.1446, 23.0208) (26.6972, 22.4561) (26.663, 21.5378) (27.0534, 21.2285) knots 0 0 0 1 2 2 2
  spline S175 degree 2 poles (27.0534, 21.2285) (27.4406, 20.9217) (28.319, 21.1554) (28.7741, 21.7297) knots 0 0 0 1 2 2 2
  spline S176 degree 2 poles (29.3885, 18.538) (29.0028, 18.8909) (28.9712, 19.7286) (29.4074, 20.2056) knots 0 0 0 1 2 2 2
  line L104 (29.4074, 20.2056) -> (30.8327, 21.7639)
  line L105 (30.8327, 21.7639) -> (30.5137, 22.0557)
  line L106 (30.5137, 22.0557) -> (30.8721, 22.4475)
  line L107 (30.8721, 22.4475) -> (31.1911, 22.1558)
  line L108 (31.1911, 22.1558) -> (31.9301, 22.9639)
  line L109 (31.9301, 22.9639) -> (32.404, 22.5304)
  line L110 (32.404, 22.5304) -> (31.665, 21.7224)
  line L111 (31.665, 21.7224) -> (32.5368, 20.925)
  line L112 (32.5368, 20.925) -> (32.1784, 20.5331)
  line L113 (32.1784, 20.5331) -> (31.3066, 21.3305)
  line L114 (31.3066, 21.3305) -> (30.0813, 19.9909)
  spline S177 degree 2 poles (30.0813, 19.9909) (29.8869, 19.7782) (29.6881, 19.5304) (29.6481, 19.3829) knots 0 0 0 1 2 2 2
  spline S178 degree 2 poles (29.6481, 19.3829) (29.61, 19.256) (29.7208, 18.9928) (29.8849, 18.8428) knots 0 0 0 1 2 2 2
  spline S179 degree 2 poles (29.8849, 18.8428) (30.0003, 18.7372) (30.2799, 18.6098) (30.3479, 18.5866) knots 0 0 0 1 2 2 2
  line L115 (30.3479, 18.5866) -> (30.3753, 18.5616)
  line L116 (30.3753, 18.5616) -> (29.9863, 18.1363)
  spline S180 degree 2 poles (29.9863, 18.1363) (29.8193, 18.2221) (29.507, 18.4297) (29.3885, 18.538) knots 0 0 0 1 2 2 2
  line L117 (30.7554, 17.308) -> (30.3017, 17.7625)
  line L118 (30.3017, 17.7625) -> (32.9996, 20.4556)
  line L119 (32.9996, 20.4556) -> (33.4533, 20.0011)
  line L120 (33.4533, 20.0011) -> (30.7554, 17.308)
  line L121 (33.934, 20.417) -> (33.4192, 20.9326)
  line L122 (33.4192, 20.9326) -> (33.8912, 21.4038)
  line L123 (33.8912, 21.4038) -> (34.406, 20.8881)
  line L124 (34.406, 20.8881) -> (33.934, 20.417)
  spline S181 degree 2 poles (32.3634, 15.451) (32.1002, 15.7458) (31.8454, 16.3959) (31.8734, 16.7354) knots 0 0 0 1 2 2 2
  spline S182 degree 2 poles (31.8734, 16.7354) (31.8983, 17.0722) (32.2844, 17.7647) (32.6591, 18.0992) knots 0 0 0 1 2 2 2
  spline S183 degree 2 poles (32.6591, 18.0992) (33.0337, 18.4336) (33.7585, 18.7221) (34.0936, 18.7177) knots 0 0 0 1 2 2 2
  spline S184 degree 2 poles (34.0936, 18.7177) (34.4317, 18.716) (35.0782, 18.3937) (35.3359, 18.1051) knots 0 0 0 1 2 2 2
  spline S185 degree 2 poles (35.3359, 18.1051) (35.5443, 17.8717) (35.8016, 17.3177) (35.8664, 17.0721) knots 0 0 0 1 2 2 2
  line L125 (35.8664, 17.0721) -> (35.329, 16.5922)
  line L126 (35.329, 16.5922) -> (35.3043, 16.6199)
  spline S186 degree 2 poles (35.3043, 16.6199) (35.3007, 16.7105) (35.2687, 16.9689) (35.2256, 17.1346) knots 0 0 0 1 2 2 2
  spline S187 degree 2 poles (35.2256, 17.1346) (35.1843, 17.2798) (35.0197, 17.6186) (34.9101, 17.7414) knots 0 0 0 1 2 2 2
  spline S188 degree 2 poles (34.9101, 17.7414) (34.5783, 18.113) (33.6133, 18.0626) (33.1005, 17.6048) knots 0 0 0 1 2 2 2
  spline S189 degree 2 poles (33.1005, 17.6048) (32.6, 17.1578) (32.4273, 16.22) (32.7728, 15.8331) knots 0 0 0 1 2 2 2
  spline S190 degree 2 poles (32.7728, 15.8331) (32.9812, 15.5997) (33.553, 15.3487) (33.8488, 15.3203) knots 0 0 0 1 2 2 2
  line L127 (33.8488, 15.3203) -> (33.8734, 15.2927)
  line L128 (33.8734, 15.2927) -> (33.336, 14.8128)
  spline S191 degree 2 poles (33.336, 14.8128) (33.2392, 14.8533) (32.9521, 14.9833) (32.8538, 15.0501) knots 0 0 0 1 2 2 2
  spline S192 degree 2 poles (32.8538, 15.0501) (32.7073, 15.14) (32.4977, 15.3006) (32.3634, 15.451) knots 0 0 0 1 2 2 2
  spline S193 degree 2 poles (34.0936, 13.3402) (33.8602, 13.6437) (33.6193, 14.2946) (33.5777, 14.5378) knots 0 0 0 1 2 2 2
  line L129 (33.5777, 14.5378) -> (34.1487, 14.977)
  line L130 (34.1487, 14.977) -> (34.1688, 14.9509)
  spline S194 degree 2 poles (34.1688, 14.9509) (34.1668, 14.8455) (34.1783, 14.5739) (34.2227, 14.3743) knots 0 0 0 1 2 2 2
  spline S195 degree 2 poles (34.2227, 14.3743) (34.2586, 14.1994) (34.4082, 13.8159) (34.5362, 13.6494) knots 0 0 0 1 2 2 2
  spline S196 degree 2 poles (34.5362, 13.6494) (34.629, 13.5287) (34.8978, 13.294) (34.9937, 13.2639) knots 0 0 0 1 2 2 2
  spline S197 degree 2 poles (34.9937, 13.2639) (35.1285, 13.2169) (35.3341, 13.24) (35.4776, 13.3504) knots 0 0 0 1 2 2 2
  spline S198 degree 2 poles (35.4776, 13.3504) (35.6571, 13.4885) (35.6925, 13.8273) (35.5613, 14.1263) knots 0 0 0 1 2 2 2
  spline S199 degree 2 poles (35.5613, 14.1263) (35.5088, 14.2417) (35.3331, 14.6052) (35.2661, 14.7666) knots 0 0 0 1 2 2 2
  spline S200 degree 2 poles (35.2661, 14.7666) (35.1013, 15.1903) (35.278, 15.8248) (35.5749, 16.0532) knots 0 0 0 1 2 2 2
  spline S201 degree 2 poles (35.5749, 16.0532) (35.9861, 16.3694) (36.9728, 16.1467) (37.3643, 15.6377) knots 0 0 0 1 2 2 2
  spline S202 degree 2 poles (37.3643, 15.6377) (37.5575, 15.3864) (37.8251, 14.782) (37.8635, 14.5363) knots 0 0 0 1 2 2 2
  line L131 (37.8635, 14.5363) -> (37.3185, 14.1171)
  line L132 (37.3185, 14.1171) -> (37.2984, 14.1432)
  spline S203 degree 2 poles (37.2984, 14.1432) (37.3045, 14.4595) (37.1175, 15.074) (36.9293, 15.3187) knots 0 0 0 1 2 2 2
  spline S204 degree 2 poles (36.9293, 15.3187) (36.736, 15.57) (36.2579, 15.7527) (36.0458, 15.5896) knots 0 0 0 1 2 2 2
  spline S205 degree 2 poles (36.0458, 15.5896) (35.8533, 15.4415) (35.8254, 15.0929) (35.9423, 14.8193) knots 0 0 0 1 2 2 2
  spline S206 degree 2 poles (35.9423, 14.8193) (35.9983, 14.6857) (36.1554, 14.3599) (36.2375, 14.1789) knots 0 0 0 1 2 2 2
  spline S207 degree 2 poles (36.2375, 14.1789) (36.4086, 13.7809) (36.2813, 13.1428) (35.9452, 12.8843) knots 0 0 0 1 2 2 2
  spline S208 degree 2 poles (35.9452, 12.8843) (35.7494, 12.7337) (35.2856, 12.6211) (35.0429, 12.6733) knots 0 0 0 1 2 2 2
  spline S209 degree 2 poles (35.0429, 12.6733) (34.7861, 12.7303) (34.3321, 13.0302) (34.0936, 13.3402) knots 0 0 0 1 2 2 2
  point P0 (0, 0)
  point P1 (39.8865, 3.0773)
  point P2 (-39.8865, 3.0773)
  dimension "d64" = 0
  constraints: 4 end point, 2 point on circle, 1 centre point, 1 collinear, 1 horizontal, 1 point on line, 1 other
  measures "d64" distance between parallel lines of L2 L3
extrude "Extrusion12" cut sketch "Sketch16" against normal blind 1.5875
equation "\"d56\" = d55"
body "Solid2"
